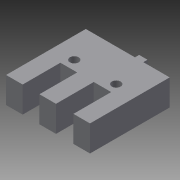
# Autodesk Inventor part: endstop
Saved by Autodesk Inventor 2014 (Build 180170000, 170)
## iProperties
Created: 2014-02-17
Part Number: endstop
Material: Generic
Document SubType Name: Modeling
Designer: stephen
Density: 1 g/cm^3
Appearance: Default
Author: stephen
Autodesk Inventor part; units mm, degrees
ref_plane "YZ Plane" through (0, 0, 0) normal (1, 0, 0) x (0, 1, 0)
ref_plane "XZ Plane" through (0, 0, 0) normal (0, 1, 0) x (-1, 0, 0)
ref_plane "XY Plane" through (0, 0, 0) normal (0, 0, 1) x (1, 0, 0)
sketch "Sketch1" plane through (0, 0, 0) normal (0, 0, 1) x (1, 0, 0)
  line L0 (20, 0) -> (20, 10)
  line L1 (20, 10) -> (0, 10)
  line L2 (0, 10) -> (0, 0)
  circle A0 centre (5, 2.25) radius 1.05
  circle A1 centre (15, 2.25) radius 1.05
  line L3 (20, 0) -> (20, -9)
  line L4 (0, -9) -> (0, 0)
  line L5 (3.95, 0) -> (3.95, -9)
  line L6 (16.05, 0) -> (16.05, -9)
  line L7 (7.95, 0) -> (7.95, -9)
  line L8 (7.95, -9) -> (11.9, -9)
  line L9 (11.9, -9) -> (11.9, 0)
  line L10 (3.95, 0) -> (7.95, 0)
  line L11 (11.9, 0) -> (16.05, 0)
  line L12 (3.95, 0) -> (7.95, 0)
  line L13 (11.9, 0) -> (16.05, 0)
  line L14 (3.95, -9) -> (0, -9)
  line L15 (20, -9) -> (16.05, -9)
  line L16 (11.9, -9) -> (7.95, -9)
  line L17 (0, -9) -> (0, 10)
  line L18 (20, 10) -> (0, 10)
  line L19 (20, 10) -> (20, -9)
  line L20 (20, -9) -> (16.05, -9)
  line L21 (16.05, -9) -> (16.05, 0)
  line L22 (16.05, 0) -> (11.9, 0)
  line L23 (11.9, -9) -> (7.95, -9)
  line L24 (7.95, -9) -> (7.95, 0)
  line L25 (7.95, 0) -> (3.95, 0)
  dimension "d0" = 20
  dimension "d1" = 10
  dimension "d2" = 2.1
  dimension "d3" = 2.1
  dimension "d4" = 5
  dimension "d5" = 5
  dimension "d12" = 9
  dimension "d13" = 3.95
  dimension "d14" = 4
  constraints: 52 end point, 15 perpendicular, 11 parallel, 5 collinear, 4 horizontal, 2 centre point
  measures "d0" distance of L1.end L0.end
  measures "d1" distance of L0.end L0.start
  measures "d2" diameter of A1
  measures "d3" diameter of A0
  measures "d4" distance from line of L0 A1.centre
  measures "d5" distance from line of L2 A0.centre
  measures "d12" distance of L3.start L3.end
  measures "d13" distance of L7.end L8.end
  measures "d14" distance between parallel lines of L7 L5
extrude "Extrusion3" add sketch "Sketch1" along normal blind 6.2
sketch "Sketch3" plane through (0, 10, 0) normal (0, 1, 0) x (1, 0, 0)
  line L0 (20, 0) -> (0, 0) projected
  line L1 (20, -6.2) -> (0, -6.2) projected
  line L2 (20, 0) -> (20, -6.2) projected
  line L3 (14, 0) -> (14, -6.2)
  line L4 (12, 0) -> (12, -6.2)
  dimension "d17" = 6
  dimension "d18" = 2
  constraints: 4 end point, 4 point on line, 2 perpendicular
  measures "d17" distance between parallel lines of L3 L2
  measures "d18" distance between parallel lines of L4 L3
extrude "Extrusion4" add sketch "Sketch3" along normal blind 1 contours L3 L1 L4 L0
body "Solid2"
